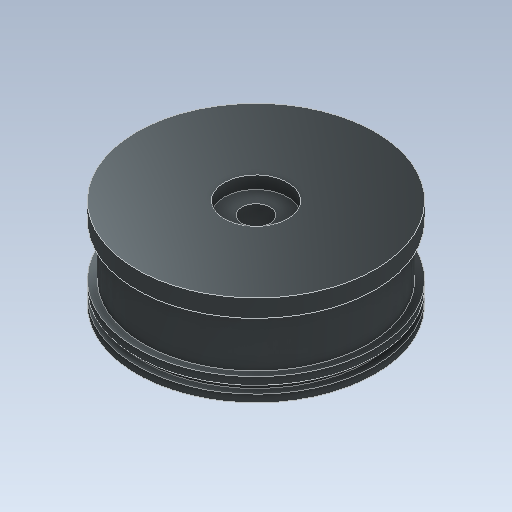
# Autodesk Inventor part: Верхняя часть поршня_CPY
Saved by Autodesk Inventor 2021 (Build 250183000, 183)
## iProperties
Created: 2020-10-24
Part Number: Верхняя часть поршня_CPY
Material: Чугун, серый
Document SubType Name: Modeling
Designer: Тимоха
Mass: 61164.2 g
Surface Area: 6102.27 cm^2
Volume: 8554.43 cm^3
Density: 7.15 g/cm^3
Appearance: Чугун серый
Author: Тимоха
Autodesk Inventor part; units mm, degrees
ref_plane "YZ Plane" through (0, 0, 0) normal (1, 0, 0) x (0, 1, 0)
ref_plane "XZ Plane" through (0, 0, 0) normal (0, 1, 0) x (-1, 0, 0)
ref_plane "XY Plane" through (0, 0, 0) normal (0, 0, 1) x (1, 0, 0)
sketch "Эскиз1" plane through (0, 0, 0) normal (0, 0, 1) x (1, 0, 0)
  line L0 (49.9998, 0) -> (189, 0)
  line L1 (189, 0) -> (189, -28)
  line L2 (189, -28) -> (178, -28)
  line L3 (178, -28) -> (178, -108)
  line L4 (178, -108) -> (189, -108)
  line L5 (150.5518, -43) -> (70.9998, -43)
  line L6 (54.9998, -59) -> (54.9998, -152)
  line L7 (24.9998, -84) -> (22.4998, -84)
  line L8 (22.4998, -84) -> (22.4998, -20)
  line L9 (22.4998, -20) -> (49.9998, -20)
  line L10 (49.9998, -20) -> (49.9998, 0)
  arc A0 (70.9998, -43) -> (54.9998, -59) centre (70.9998, -59) ccw
  line L11 (0, 0) -> (0, 25.6698)
  line L12 (189, -108) -> (189, -120)
  line L13 (189, -144) -> (169, -144)
  line L14 (169, -144) -> (169, -152)
  line L15 (189, -144) -> (189, -132)
  line L16 (189, -132) -> (178, -132)
  line L17 (178, -132) -> (178, -120)
  line L18 (178, -120) -> (189, -120)
  line L19 (189, -108) -> (189, -120)
  line L20 (160, -152) -> (160, -106)
  line L21 (34.9998, -144) -> (34.9998, -94)
  line L22 (169, -152) -> (160, -152)
  line L23 (54.9998, -152) -> (39.9998, -152)
  line L24 (39.9998, -152) -> (39.9998, -144)
  line L25 (39.9998, -144) -> (34.9998, -144)
  arc A1 (34.9998, -94) -> (24.9998, -84) centre (24.9998, -94) ccw
  line L26 (160, -106) -> (166.391, -61.2627)
  arc A2 (166.391, -61.2627) -> (150.5518, -43) centre (150.5518, -59) ccw
  point P0 (54.9998, -43)
  point P1 (34.9998, -98)
  dimension "d0" = 189
  dimension "d1" = 28
  dimension "d2" = 11
  dimension "d3" = 80
  dimension "d17" = 64
  dimension "d18" = 27.5
  dimension "d24" = 16
  dimension "d29" = 20
  dimension "d30" = 8
  dimension "d31" = 12
  dimension "d32" = 11
  dimension "d33" = 12
  dimension "d34" = 12
  dimension "d35" = 46
  dimension "d36" = 93
  dimension "d37" = 46
  dimension "d38" = 15
  dimension "d39" = 20
  dimension "d40" = 5
  dimension "d41" = 8
  dimension "d42" = 10
  dimension "d43" = 9
  dimension "d44" = 169
  dimension "d45" = 16
  constraints: 54 end point, 14 perpendicular, 6 point on circle, 6 tangent, 5 vertical, 4 horizontal, 4 point on line, 3 centre point, 1 collinear
  measures "d0" distance of L11.start L0.end
  measures "d1" distance of L0.end L1.end
  measures "d2" distance of L1.end L2.end
  measures "d3" distance of L2.end L3.end
  measures "d17" distance of L7.end L8.end
  measures "d18" distance of L8.end L9.end
  measures "d24" radius of A0
  measures "d29" distance of L13.start L13.end
  measures "d30" distance of L13.end L14.end
  measures "d31" distance of L15.end L13.start
  measures "d32" distance of L15.end L16.end
  measures "d33" distance of L16.end L17.end
  measures "d34" distance of L4.end L12.end
  measures "d35" distance of L20.start L20.end
  measures "d36" distance of L6.start L6.end
  measures "d37" distance of L21.start point (35, -98)
  measures "d38" distance of L6.end L23.end
  measures "d39" distance of L9.end L0.start
  measures "d40" distance of L24.end L21.start
  measures "d41" distance of L23.end L24.end
  measures "d42" radius of A1
  measures "d43" distance of L14.end L20.start
  measures "d44" distance from line of L14 L11.start
  measures "d45" radius of A2
revolve "Вращение1" add sketch "Эскиз1" angle 360 about axis through (0, 0, 0) along (0, 1, 0)
